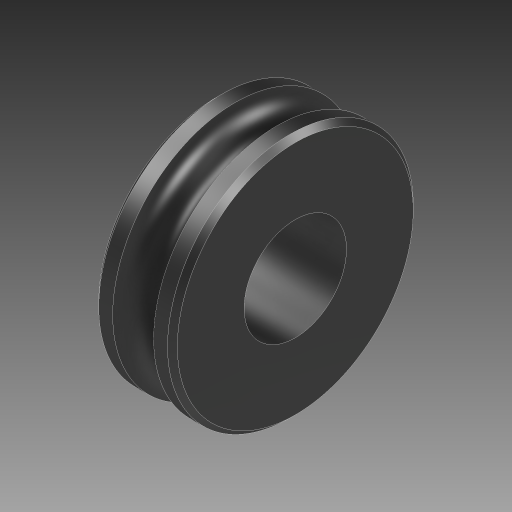
# Autodesk Inventor part: Custom Cascade Bearing Pulley
Saved by Autodesk Inventor 2024 (Build 280153000, 153)
## iProperties
Created: 2023-05-06
Part Number: Custom Cascade Bearing Pulley
Material: Aluminum
Document SubType Name: Modeling
Designer: Max Boord
Mass: 26.0738 g
Surface Area: 41.5048 cm^2
Volume: 9.65698 cm^3
Density: 2.7 g/cm^3
Appearance: Glossy - Black
Author: Max Boord
Autodesk Inventor part; units mm, degrees
ref_plane "YZ Plane" through (0, 0, 0) normal (1, 0, 0) x (0, 1, 0)
ref_plane "XZ Plane" through (0, 0, 0) normal (0, 1, 0) x (-1, 0, 0)
ref_plane "XY Plane" through (0, 0, 0) normal (0, 0, 1) x (1, 0, 0)
sketch "Sketch1" plane through (0, 0, 0) normal (0, 0, 1) x (1, 0, 0)
  line L0 (0, 0) -> (0, 13.9169) construction
  arc A0 (-3.175, 19.05) -> (3.175, 19.05) centre (0, 19.05) ccw
  line L1 (-3.175, 19.05) -> (-5.334, 19.05)
  line L2 (3.175, 19.05) -> (5.334, 19.05)
  line L3 (6.096, 18.288) -> (6.096, 7.9375)
  line L4 (6.096, 7.9375) -> (-6.096, 7.9375)
  line L5 (-6.096, 7.9375) -> (-6.096, 18.288)
  line L6 (0, 0) -> (7.2482, 0) construction
  line L7 (-5.334, 19.05) -> (-6.096, 18.288)
  line L8 (5.334, 19.05) -> (6.096, 18.288)
  point P0 (-6.096, 19.05)
  point P1 (6.096, 19.05)
  dimension "d0" = 6.35
  dimension "d1" = 15.875
  dimension "d2" = 38.1
  dimension "d3" = 12.192
  dimension "d4" = 0.762
  dimension "d5" = 0.762
  dimension "d6" = 0.762
  dimension "d7" = 0.762
  constraints: 18 end point, 5 point on line, 3 horizontal, 2 collinear, 2 perpendicular, 2 point on circle, 2 vertical, 1 centre point, 1 horizontal alignment
  measures "d0" diameter of A0
  measures "d1" diameter of L4 L6
  measures "d2" diameter of L2 L6
  measures "d3" distance between parallel lines of L3 L5
  measures "d4" distance of L1.end point (-6.096, 19.05)
  measures "d5" distance of L5.end point (-6.096, 19.05)
  measures "d6" distance of L2.end point (6.096, 19.05)
  measures "d7" distance of L3.start point (6.096, 19.05)
revolve "Revolution1" add sketch "Sketch1" angle 360 about axis through (0, 0, 0) along (1, 0, 0)
equation "\"d5\" = d4"
equation "\"d6\" = d4"
equation "\"d7\" = d6"
body "Solid1"
